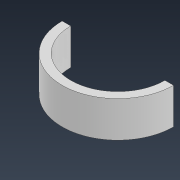
# Autodesk Inventor part: Panewka środkowa wału korbowego
Saved by Autodesk Inventor 2022 (Build 260153000, 153)
## iProperties
Created: 2023-05-24
Part Number: Panewka środkowa wału korbowego
Material: Generic
Document SubType Name: Modeling
Designer: wikto
Density: 1 g/cm^3
Appearance: Default
Author: wikto
Autodesk Inventor part; units mm, degrees
ref_plane "YZ Plane" through (0, 0, 0) normal (1, 0, 0) x (0, 1, 0)
ref_plane "XZ Plane" through (0, 0, 0) normal (0, 1, 0) x (-1, 0, 0)
ref_plane "XY Plane" through (0, 0, 0) normal (0, 0, 1) x (1, 0, 0)
sketch "Sketch1" plane through (0, 0, 0) normal (0, 1, 0) x (-1, 0, 0)
  circle A0 centre (0, 0) radius 27.5
  circle A1 centre (0, 0) radius 32.5
  line L0 (32.5, 0) -> (-32.5, 0)
  point P0 (27.5, 0)
  point P1 (-27.5, 0)
  dimension "d0" = 55
  dimension "d1" = 65
  constraints: 2 centre point, 2 coincident, 2 end point, 2 point on circle, 1 horizontal, 1 horizontal alignment
  measures "d0" diameter of A0
  measures "d1" diameter of A1
extrude "Extrusion1" add sketch "Sketch1" along normal blind 21 contours A0 L0 A1 picked at (28.2277, 11.887)
body "Solid1"
